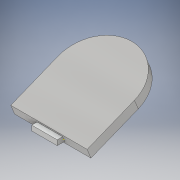
# Autodesk Inventor part: Aparture_door
Saved by Autodesk Inventor 2018 (Build 220112000, 112)
## iProperties
Created: 2021-02-20
Part Number: Aparture_door
Material: Generic
Document SubType Name: Modeling
Designer: Patel
Density: 1 g/cm^3
Appearance: Default
Author: Patel
Autodesk Inventor part; units mm, degrees
ref_plane "YZ Plane" through (0, 0, 0) normal (1, 0, 0) x (0, 1, 0)
ref_plane "XZ Plane" through (0, 0, 0) normal (0, 1, 0) x (-1, 0, 0)
sketch "Sketch1" plane through (0, 0, 0) normal (0, 0, 1) x (1, 0, 0)
  line L0 (-50, 10) -> (50, 10)
  line L1 (50, 10) -> (50, -10)
  line L2 (50, -10) -> (-50, -10)
  line L3 (-50, -10) -> (-50, 10)
  line L4 (-50, 10) -> (50, -10) construction
  line L5 (50, 10) -> (-50, -10) construction
  point P0 (0, 0)
  dimension "d0" = 100
  dimension "d1" = 20
  constraints: 12 end point, 2 midpoint, 2 parallel, 1 horizontal, 1 perpendicular
  measures "d0" distance of L1.end L2.end
  measures "d1" distance of L0.end L1.end
extrude "Extrusion1" add sketch "Sketch1" along normal mid plane 50
sketch "Sketch2" plane through (0, 0, 0) normal (0, 0, 1) x (1, 0, 0)
  point P0 (0, 0)
ref_plane "Work Plane1" through (50, -10, 25) normal (0, 0.9285, 0.3714) x (1, 0, 0)
sketch "Sketch3" plane through (50, -10, 25) normal (1, 0, 0) x (0, 0, -1)
  point P0 (25, 10)
sketch "Sketch4" plane through (50, -10, 25) normal (0, 0.9285, 0.3714) x (1, 0, 0)
  line L0 (0, 0) -> (0, 46.4238) construction
  line L1 (0, 26.9258) -> (-109.9781, 26.9258) construction
  line L2 (-200, 26.9258) -> (100, 26.9258)
  line L3 (100, 26.9258) -> (100, 226.9258)
  line L4 (-200, 226.9258) -> (-200, 26.9258)
  arc A0 (100, 226.9258) -> (-200, 226.9258) centre (-50, 226.9258) ccw
  point P0 (-50, 26.9258)
  dimension "d4" = 300
  dimension "d5" = 200
  dimension "d6" = 300
  dimension "d7" = 100
  dimension "d8" = 19.498
  dimension "d9" = 109.9781
  constraints: 9 end point, 2 horizontal, 2 point on circle, 2 point on line, 1 centre point, 1 parallel, 1 perpendicular, 1 tangent
  measures "d4" distance of L4.start L3.end
  measures "d5" distance of L3.end L2.end
  measures "d6" diameter of A0
  measures "d7" distance between parallel lines of L0 L3
  measures "d8" distance from line of L0.end L1
  measures "d9" distance from line of L1.end L0
extrude "Extrusion2" add sketch "Sketch4" along normal mid plane 40
body "Solid1"
